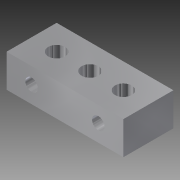
# Autodesk Inventor part: 09-0004
Saved by Autodesk Inventor 2015 SP1 (Build 190203100, 203)
## iProperties
Category: Joiner Block Kit
Company: Autodesk Inc.
Created: 2014-11-30
Part Number: 09-0004
Material: Aluminum 6061
Document SubType Name: Modeling
Designer: Matrix
Density: 2.7 g/cm^3
Appearance: Aluminum - Polished
Catalog Web Link: http://matrixrobotics.com/
Vendor: Matrix
Author: Autodesk Inc.
Autodesk Inventor part; units mm, degrees
ref_plane "YZ Plane" through (0, 0, 0) normal (1, 0, 0) x (0, 1, 0)
ref_plane "XZ Plane" through (0, 0, 0) normal (0, 1, 0) x (-1, 0, 0)
ref_plane "XY Plane" through (0, 0, 0) normal (0, 0, 1) x (1, 0, 0)
sketch "Sketch1" plane through (0, 0, 0) normal (0, 1, 0) x (-1, 0, 0)
  line L0 (0, 0) -> (7.9, 0)
  line L1 (7.9, 0) -> (7.9, -28)
  line L2 (7.9, -28) -> (0, -28)
  line L3 (0, -28) -> (0, 0)
  dimension "d0" = 7.9
  dimension "d1" = 28
  constraints: 8 end point, 2 parallel, 1 horizontal, 1 perpendicular
  measures "d0" distance of L1.end L2.end
  measures "d1" distance of L0.end L1.end
extrude "Extrusion1" add sketch "Sketch1" against normal blind 12
sketch "Sketch2" plane through (0, 0, 0) normal (0, 1, 0) x (1, 0, 0)
  line L0 (0, 0) -> (-7.9, 0) projected
  line L1 (-7.9, 28) -> (0, 28) projected
  point P0 (-4.043, 6)
  point P1 (-4.043, 22)
  dimension "d4" = 6
  dimension "d5" = 6
  constraints: 1 vertical alignment
  measures "d4" distance from line of point (-4.043, 6) L0
  measures "d5" distance from line of point (-4.043, 22) L1
hole "Hole1" at (-4.043, 0, -6) at (-4.043, 0, -22) direction (0, -1, 0) diameter 3 end through all
sketch "Sketch3" plane through (-7.9, 0, -28) normal (-1, 0, 0) x (0, 0, 1)
  line L0 (28, 0) -> (28, -12) projected
  point P0 (22, -6)
  point P1 (14, -6)
  point P2 (6, -6)
  point P3 (28, -6)
  dimension "d13" = 6
  dimension "d14" = 8
  dimension "d15" = 8
  constraints: 3 horizontal alignment, 1 midpoint
  measures "d13" distance from line of point (22, -6) L0
  measures "d14" distance of point (14, -6) point (22, -6)
  measures "d15" distance of point (6, -6) point (14, -6)
hole "Hole2" at (-7.9, -6, -6) at (-7.9, -6, -14) at (-7.9, -6, -22) direction (1, 0, 0) diameter 4 end through all
equation "\"d15\" = d14"
body "Solid1"
